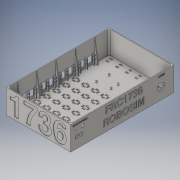
# Autodesk Inventor part: main_enclosure
Saved by Autodesk Inventor 2016 (Build 200138000, 138)
## iProperties
Created: 2015-08-24
Part Number: main_enclosure
Material: Generic
Document SubType Name: Modeling
Designer: Chris Gerth
Density: 1 g/cm^3
Appearance: Default
Sheet Metal Rule: Default
Author: Chris Gerth
Autodesk Inventor part; units mm, degrees
(part 1 of 3)
ref_plane "YZ Plane" through (0, 0, 0) normal (1, 0, 0) x (0, 1, 0)
ref_plane "XZ Plane" through (0, 0, 0) normal (0, 1, 0) x (-1, 0, 0)
ref_plane "XY Plane" through (0, 0, 0) normal (0, 0, 1) x (1, 0, 0)
sketch "Sketch1" plane through (0, 0, 0) normal (0, 1, 0) x (-1, 0, 0)
  line L0 (127, 203.2) -> (-127, 203.2)
  line L1 (-127, 203.2) -> (-127, -203.2)
  line L2 (-127, -203.2) -> (127, -203.2)
  line L3 (127, -203.2) -> (127, 203.2)
  line L4 (117.475, 184.15) -> (112.7125, 184.15)
  line L5 (112.7125, 184.15) -> (112.7125, 174.625)
  line L6 (112.7125, 174.625) -> (117.475, 174.625)
  line L7 (117.475, 174.625) -> (117.475, 184.15)
  line L8 (109.5375, 174.625) -> (100.0125, 174.625)
  line L9 (100.0125, 174.625) -> (100.0125, 169.8625)
  line L10 (100.0125, 169.8625) -> (109.5375, 169.8625)
  line L11 (109.5375, 169.8625) -> (109.5375, 174.625)
  line L12 (96.8375, 174.625) -> (92.0652, 174.625)
  line L13 (92.0652, 174.625) -> (92.0652, 184.2167)
  line L14 (92.0652, 184.2167) -> (96.8375, 184.2167)
  line L15 (96.8375, 184.2167) -> (96.8375, 174.625)
  line L16 (109.5375, 184.15) -> (100.0125, 184.15)
  line L17 (100.0125, 184.15) -> (100.0125, 188.9125)
  line L18 (100.0125, 188.9125) -> (109.5375, 188.9125)
  line L19 (109.5375, 188.9125) -> (109.5375, 184.15)
  line L20 (112.7125, 146.05) -> (112.7125, 136.525)
  line L21 (117.475, 146.05) -> (112.7125, 146.05)
  line L22 (112.7125, 136.525) -> (117.475, 136.525)
  line L23 (117.475, 136.525) -> (117.475, 146.05)
  line L24 (109.5375, 131.7625) -> (109.5375, 136.525)
  line L25 (109.5375, 150.8125) -> (109.5375, 146.05)
  line L26 (100.0125, 136.525) -> (100.0125, 131.7625)
  line L27 (100.0125, 131.7625) -> (109.5375, 131.7625)
  line L28 (100.0125, 146.05) -> (100.0125, 150.8125)
  line L29 (100.0125, 150.8125) -> (109.5375, 150.8125)
  line L30 (109.5375, 136.525) -> (100.0125, 136.525)
  line L31 (109.5375, 146.05) -> (100.0125, 146.05)
  line L32 (96.8375, 146.1167) -> (96.8375, 136.525)
  line L33 (96.8375, 136.525) -> (92.0652, 136.525)
  line L34 (92.0652, 136.525) -> (92.0652, 146.1167)
  line L35 (92.0652, 146.1167) -> (96.8375, 146.1167)
  line L36 (112.7125, 107.95) -> (112.7125, 98.425)
  line L37 (117.475, 107.95) -> (112.7125, 107.95)
  line L38 (112.7125, 98.425) -> (117.475, 98.425)
  line L39 (117.475, 98.425) -> (117.475, 107.95)
  line L40 (109.5375, 93.6625) -> (109.5375, 98.425)
  line L41 (109.5375, 112.7125) -> (109.5375, 107.95)
  line L42 (100.0125, 98.425) -> (100.0125, 93.6625)
  line L43 (100.0125, 93.6625) -> (109.5375, 93.6625)
  line L44 (100.0125, 107.95) -> (100.0125, 112.7125)
  line L45 (100.0125, 112.7125) -> (109.5375, 112.7125)
  line L46 (109.5375, 98.425) -> (100.0125, 98.425)
  line L47 (109.5375, 107.95) -> (100.0125, 107.95)
  line L48 (96.8375, 108.0167) -> (96.8375, 98.425)
  line L49 (96.8375, 98.425) -> (92.0652, 98.425)
  line L50 (92.0652, 98.425) -> (92.0652, 108.0167)
  line L51 (92.0652, 108.0167) -> (96.8375, 108.0167)
  line L52 (112.7125, 69.85) -> (112.7125, 60.325)
  line L53 (117.475, 69.85) -> (112.7125, 69.85)
  line L54 (112.7125, 60.325) -> (117.475, 60.325)
  line L55 (117.475, 60.325) -> (117.475, 69.85)
  line L56 (109.5375, 55.5625) -> (109.5375, 60.325)
  line L57 (109.5375, 74.6125) -> (109.5375, 69.85)
  line L58 (100.0125, 60.325) -> (100.0125, 55.5625)
  line L59 (100.0125, 55.5625) -> (109.5375, 55.5625)
  line L60 (100.0125, 69.85) -> (100.0125, 74.6125)
  line L61 (100.0125, 74.6125) -> (109.5375, 74.6125)
  line L62 (109.5375, 60.325) -> (100.0125, 60.325)
  line L63 (109.5375, 69.85) -> (100.0125, 69.85)
  line L64 (96.8375, 69.9167) -> (96.8375, 60.325)
  line L65 (96.8375, 60.325) -> (92.0652, 60.325)
  line L66 (92.0652, 60.325) -> (92.0652, 69.9167)
  line L67 (92.0652, 69.9167) -> (96.8375, 69.9167)
  line L68 (112.7125, 31.75) -> (112.7125, 22.225)
  line L69 (117.475, 31.75) -> (112.7125, 31.75)
  line L70 (112.7125, 22.225) -> (117.475, 22.225)
  line L71 (117.475, 22.225) -> (117.475, 31.75)
  line L72 (109.5375, 17.4625) -> (109.5375, 22.225)
  line L73 (109.5375, 36.5125) -> (109.5375, 31.75)
  line L74 (100.0125, 22.225) -> (100.0125, 17.4625)
  line L75 (100.0125, 17.4625) -> (109.5375, 17.4625)
  line L76 (100.0125, 31.75) -> (100.0125, 36.5125)
  line L77 (100.0125, 36.5125) -> (109.5375, 36.5125)
  line L78 (109.5375, 22.225) -> (100.0125, 22.225)
  line L79 (109.5375, 31.75) -> (100.0125, 31.75)
  line L80 (96.8375, 31.8167) -> (96.8375, 22.225)
  line L81 (96.8375, 22.225) -> (92.0652, 22.225)
  line L82 (92.0652, 22.225) -> (92.0652, 31.8167)
  line L83 (92.0652, 31.8167) -> (96.8375, 31.8167)
  line L84 (112.7125, -6.35) -> (112.7125, -15.875)
  line L85 (117.475, -6.35) -> (112.7125, -6.35)
  line L86 (112.7125, -15.875) -> (117.475, -15.875)
  line L87 (117.475, -15.875) -> (117.475, -6.35)
  line L88 (109.5375, -20.6375) -> (109.5375, -15.875)
  line L89 (109.5375, -1.5875) -> (109.5375, -6.35)
  line L90 (100.0125, -15.875) -> (100.0125, -20.6375)
  line L91 (100.0125, -20.6375) -> (109.5375, -20.6375)
  line L92 (100.0125, -6.35) -> (100.0125, -1.5875)
  line L93 (100.0125, -1.5875) -> (109.5375, -1.5875)
  line L94 (109.5375, -15.875) -> (100.0125, -15.875)
  line L95 (109.5375, -6.35) -> (100.0125, -6.35)
  line L96 (96.8375, -6.2833) -> (96.8375, -15.875)
  line L97 (96.8375, -15.875) -> (92.0652, -15.875)
  line L98 (92.0652, -15.875) -> (92.0652, -6.2833)
  line L99 (92.0652, -6.2833) -> (96.8375, -6.2833)
  line L100 (112.7125, -44.45) -> (112.7125, -53.975)
  line L101 (117.475, -44.45) -> (112.7125, -44.45)
  line L102 (112.7125, -53.975) -> (117.475, -53.975)
  line L103 (117.475, -53.975) -> (117.475, -44.45)
  line L104 (109.5375, -58.7375) -> (109.5375, -53.975)
  line L105 (109.5375, -39.6875) -> (109.5375, -44.45)
  line L106 (100.0125, -53.975) -> (100.0125, -58.7375)
  line L107 (100.0125, -58.7375) -> (109.5375, -58.7375)
  line L108 (100.0125, -44.45) -> (100.0125, -39.6875)
  line L109 (100.0125, -39.6875) -> (109.5375, -39.6875)
  line L110 (109.5375, -53.975) -> (100.0125, -53.975)
  line L111 (109.5375, -44.45) -> (100.0125, -44.45)
  line L112 (96.8375, -44.3833) -> (96.8375, -53.975)
  line L113 (96.8375, -53.975) -> (92.0652, -53.975)
  line L114 (92.0652, -53.975) -> (92.0652, -44.3833)
  line L115 (92.0652, -44.3833) -> (96.8375, -44.3833)
  line L116 (74.6125, 184.15) -> (74.6125, 174.625)
  line L117 (79.375, 184.15) -> (74.6125, 184.15)
  line L118 (74.6125, 174.625) -> (79.375, 174.625)
  line L119 (79.375, 174.625) -> (79.375, 184.15)
  line L120 (71.4375, 169.8625) -> (71.4375, 174.625)
  line L121 (71.4375, 188.9125) -> (71.4375, 184.15)
  line L122 (61.9125, 174.625) -> (61.9125, 169.8625)
  line L123 (61.9125, 169.8625) -> (71.4375, 169.8625)
  line L124 (61.9125, 184.15) -> (61.9125, 188.9125)
  line L125 (61.9125, 188.9125) -> (71.4375, 188.9125)
  line L126 (71.4375, 174.625) -> (61.9125, 174.625)
  line L127 (71.4375, 184.15) -> (61.9125, 184.15)
  line L128 (58.7375, 184.2167) -> (58.7375, 174.625)
  line L129 (58.7375, 174.625) -> (53.9652, 174.625)
  line L130 (53.9652, 174.625) -> (53.9652, 184.2167)
  line L131 (53.9652, 184.2167) -> (58.7375, 184.2167)
  line L132 (74.6125, 146.05) -> (74.6125, 136.525)
  line L133 (79.375, 146.05) -> (74.6125, 146.05)
  line L134 (74.6125, 136.525) -> (79.375, 136.525)
  line L135 (79.375, 136.525) -> (79.375, 146.05)
  line L136 (71.4375, 131.7625) -> (71.4375, 136.525)
  line L137 (71.4375, 150.8125) -> (71.4375, 146.05)
  line L138 (61.9125, 136.525) -> (61.9125, 131.7625)
  line L139 (61.9125, 131.7625) -> (71.4375, 131.7625)
  line L140 (61.9125, 146.05) -> (61.9125, 150.8125)
  line L141 (61.9125, 150.8125) -> (71.4375, 150.8125)
  line L142 (71.4375, 136.525) -> (61.9125, 136.525)
  line L143 (71.4375, 146.05) -> (61.9125, 146.05)
  line L144 (58.7375, 146.1167) -> (58.7375, 136.525)
  line L145 (58.7375, 136.525) -> (53.9652, 136.525)
  line L146 (53.9652, 136.525) -> (53.9652, 146.1167)
  line L147 (53.9652, 146.1167) -> (58.7375, 146.1167)
  line L148 (74.6125, 107.95) -> (74.6125, 98.425)
  line L149 (79.375, 107.95) -> (74.6125, 107.95)
  line L150 (74.6125, 98.425) -> (79.375, 98.425)
  line L151 (79.375, 98.425) -> (79.375, 107.95)
  line L152 (71.4375, 93.6625) -> (71.4375, 98.425)
  line L153 (71.4375, 112.7125) -> (71.4375, 107.95)
  line L154 (61.9125, 98.425) -> (61.9125, 93.6625)
  line L155 (61.9125, 93.6625) -> (71.4375, 93.6625)
  line L156 (61.9125, 107.95) -> (61.9125, 112.7125)
  line L157 (61.9125, 112.7125) -> (71.4375, 112.7125)
  line L158 (71.4375, 98.425) -> (61.9125, 98.425)
  line L159 (71.4375, 107.95) -> (61.9125, 107.95)
  line L160 (58.7375, 108.0167) -> (58.7375, 98.425)
  line L161 (58.7375, 98.425) -> (53.9652, 98.425)
  line L162 (53.9652, 98.425) -> (53.9652, 108.0167)
  line L163 (53.9652, 108.0167) -> (58.7375, 108.0167)
  line L164 (74.6125, 69.85) -> (74.6125, 60.325)
  line L165 (79.375, 69.85) -> (74.6125, 69.85)
  line L166 (74.6125, 60.325) -> (79.375, 60.325)
  line L167 (79.375, 60.325) -> (79.375, 69.85)
  line L168 (71.4375, 55.5625) -> (71.4375, 60.325)
  line L169 (71.4375, 74.6125) -> (71.4375, 69.85)
  line L170 (61.9125, 60.325) -> (61.9125, 55.5625)
  line L171 (61.9125, 55.5625) -> (71.4375, 55.5625)
  line L172 (61.9125, 69.85) -> (61.9125, 74.6125)
  line L173 (61.9125, 74.6125) -> (71.4375, 74.6125)
  line L174 (71.4375, 60.325) -> (61.9125, 60.325)
  line L175 (71.4375, 69.85) -> (61.9125, 69.85)
  line L176 (58.7375, 69.9167) -> (58.7375, 60.325)
  line L177 (58.7375, 60.325) -> (53.9652, 60.325)
  line L178 (53.9652, 60.325) -> (53.9652, 69.9167)
  line L179 (53.9652, 69.9167) -> (58.7375, 69.9167)
  line L180 (74.6125, 31.75) -> (74.6125, 22.225)
  line L181 (79.375, 31.75) -> (74.6125, 31.75)
  line L182 (74.6125, 22.225) -> (79.375, 22.225)
  line L183 (79.375, 22.225) -> (79.375, 31.75)
  line L184 (71.4375, 17.4625) -> (71.4375, 22.225)
  line L185 (71.4375, 36.5125) -> (71.4375, 31.75)
  line L186 (61.9125, 22.225) -> (61.9125, 17.4625)
  line L187 (61.9125, 17.4625) -> (71.4375, 17.4625)
  line L188 (61.9125, 31.75) -> (61.9125, 36.5125)
  line L189 (61.9125, 36.5125) -> (71.4375, 36.5125)
  line L190 (71.4375, 22.225) -> (61.9125, 22.225)
  line L191 (71.4375, 31.75) -> (61.9125, 31.75)
  line L192 (58.7375, 31.8167) -> (58.7375, 22.225)
  line L193 (58.7375, 22.225) -> (53.9652, 22.225)
  line L194 (53.9652, 22.225) -> (53.9652, 31.8167)
  line L195 (53.9652, 31.8167) -> (58.7375, 31.8167)
  line L196 (74.6125, -6.35) -> (74.6125, -15.875)
  line L197 (79.375, -6.35) -> (74.6125, -6.35)
  line L198 (74.6125, -15.875) -> (79.375, -15.875)
  line L199 (79.375, -15.875) -> (79.375, -6.35)
  line L200 (71.4375, -20.6375) -> (71.4375, -15.875)
  line L201 (71.4375, -1.5875) -> (71.4375, -6.35)
  line L202 (61.9125, -15.875) -> (61.9125, -20.6375)
  line L203 (61.9125, -20.6375) -> (71.4375, -20.6375)
  line L204 (61.9125, -6.35) -> (61.9125, -1.5875)
  line L205 (61.9125, -1.5875) -> (71.4375, -1.5875)
  line L206 (71.4375, -15.875) -> (61.9125, -15.875)
  line L207 (71.4375, -6.35) -> (61.9125, -6.35)
  line L208 (58.7375, -6.2833) -> (58.7375, -15.875)
  line L209 (58.7375, -15.875) -> (53.9652, -15.875)
  line L210 (53.9652, -15.875) -> (53.9652, -6.2833)
  line L211 (53.9652, -6.2833) -> (58.7375, -6.2833)
  line L212 (74.6125, -44.45) -> (74.6125, -53.975)
  line L213 (79.375, -44.45) -> (74.6125, -44.45)
  line L214 (74.6125, -53.975) -> (79.375, -53.975)
  line L215 (79.375, -53.975) -> (79.375, -44.45)
  line L216 (71.4375, -58.7375) -> (71.4375, -53.975)
  line L217 (71.4375, -39.6875) -> (71.4375, -44.45)
  line L218 (61.9125, -53.975) -> (61.9125, -58.7375)
  line L219 (61.9125, -58.7375) -> (71.4375, -58.7375)
  line L220 (61.9125, -44.45) -> (61.9125, -39.6875)
  line L221 (61.9125, -39.6875) -> (71.4375, -39.6875)
  line L222 (71.4375, -53.975) -> (61.9125, -53.975)
  line L223 (71.4375, -44.45) -> (61.9125, -44.45)
  line L224 (58.7375, -44.3833) -> (58.7375, -53.975)
  line L225 (58.7375, -53.975) -> (53.9652, -53.975)
  line L226 (53.9652, -53.975) -> (53.9652, -44.3833)
  line L227 (53.9652, -44.3833) -> (58.7375, -44.3833)
  line L228 (36.5125, 184.15) -> (36.5125, 174.625)
  line L229 (41.275, 184.15) -> (36.5125, 184.15)
  line L230 (36.5125, 174.625) -> (41.275, 174.625)
  line L231 (41.275, 174.625) -> (41.275, 184.15)
  line L232 (33.3375, 169.8625) -> (33.3375, 174.625)
  line L233 (33.3375, 188.9125) -> (33.3375, 184.15)
  line L234 (23.8125, 174.625) -> (23.8125, 169.8625)
  line L235 (23.8125, 169.8625) -> (33.3375, 169.8625)
  line L236 (23.8125, 184.15) -> (23.8125, 188.9125)
  line L237 (23.8125, 188.9125) -> (33.3375, 188.9125)
  line L238 (33.3375, 174.625) -> (23.8125, 174.625)
  line L239 (33.3375, 184.15) -> (23.8125, 184.15)
  line L240 (20.6375, 184.2167) -> (20.6375, 174.625)
  line L241 (20.6375, 174.625) -> (15.8652, 174.625)
  line L242 (15.8652, 174.625) -> (15.8652, 184.2167)
  line L243 (15.8652, 184.2167) -> (20.6375, 184.2167)
  line L244 (36.5125, 146.05) -> (36.5125, 136.525)
  line L245 (41.275, 146.05) -> (36.5125, 146.05)
  line L246 (36.5125, 136.525) -> (41.275, 136.525)
  line L247 (41.275, 136.525) -> (41.275, 146.05)
  line L248 (33.3375, 131.7625) -> (33.3375, 136.525)
  line L249 (33.3375, 150.8125) -> (33.3375, 146.05)
  line L250 (23.8125, 136.525) -> (23.8125, 131.7625)
  line L251 (23.8125, 131.7625) -> (33.3375, 131.7625)
  line L252 (23.8125, 146.05) -> (23.8125, 150.8125)
  line L253 (23.8125, 150.8125) -> (33.3375, 150.8125)
  line L254 (33.3375, 136.525) -> (23.8125, 136.525)
  line L255 (33.3375, 146.05) -> (23.8125, 146.05)
  line L256 (20.6375, 146.1167) -> (20.6375, 136.525)
  line L257 (20.6375, 136.525) -> (15.8652, 136.525)
  line L258 (15.8652, 136.525) -> (15.8652, 146.1167)
  line L259 (15.8652, 146.1167) -> (20.6375, 146.1167)
  line L260 (36.5125, 107.95) -> (36.5125, 98.425)
  line L261 (41.275, 107.95) -> (36.5125, 107.95)
  line L262 (36.5125, 98.425) -> (41.275, 98.425)
  line L263 (41.275, 98.425) -> (41.275, 107.95)
  line L264 (33.3375, 93.6625) -> (33.3375, 98.425)
  line L265 (33.3375, 112.7125) -> (33.3375, 107.95)
  line L266 (23.8125, 98.425) -> (23.8125, 93.6625)
  line L267 (23.8125, 93.6625) -> (33.3375, 93.6625)
  line L268 (23.8125, 107.95) -> (23.8125, 112.7125)
  line L269 (23.8125, 112.7125) -> (33.3375, 112.7125)
  line L270 (33.3375, 98.425) -> (23.8125, 98.425)
  line L271 (33.3375, 107.95) -> (23.8125, 107.95)
  line L272 (20.6375, 108.0167) -> (20.6375, 98.425)
  line L273 (20.6375, 98.425) -> (15.8652, 98.425)
  line L274 (15.8652, 98.425) -> (15.8652, 108.0167)
  line L275 (15.8652, 108.0167) -> (20.6375, 108.0167)
  line L276 (36.5125, 69.85) -> (36.5125, 60.325)
  line L277 (41.275, 69.85) -> (36.5125, 69.85)
  line L278 (36.5125, 60.325) -> (41.275, 60.325)
  line L279 (41.275, 60.325) -> (41.275, 69.85)
  line L280 (33.3375, 55.5625) -> (33.3375, 60.325)
  line L281 (33.3375, 74.6125) -> (33.3375, 69.85)
  line L282 (23.8125, 60.325) -> (23.8125, 55.5625)
  line L283 (23.8125, 55.5625) -> (33.3375, 55.5625)
  line L284 (23.8125, 69.85) -> (23.8125, 74.6125)
  line L285 (23.8125, 74.6125) -> (33.3375, 74.6125)
  line L286 (33.3375, 60.325) -> (23.8125, 60.325)
  line L287 (33.3375, 69.85) -> (23.8125, 69.85)
  line L288 (20.6375, 69.9167) -> (20.6375, 60.325)
  line L289 (20.6375, 60.325) -> (15.8652, 60.325)
  line L290 (15.8652, 60.325) -> (15.8652, 69.9167)
  line L291 (15.8652, 69.9167) -> (20.6375, 69.9167)
  line L292 (36.5125, 31.75) -> (36.5125, 22.225)
  line L293 (41.275, 31.75) -> (36.5125, 31.75)
  line L294 (36.5125, 22.225) -> (41.275, 22.225)
  line L295 (41.275, 22.225) -> (41.275, 31.75)
  line L296 (33.3375, 17.4625) -> (33.3375, 22.225)
  line L297 (33.3375, 36.5125) -> (33.3375, 31.75)
  line L298 (23.8125, 22.225) -> (23.8125, 17.4625)
  line L299 (23.8125, 17.4625) -> (33.3375, 17.4625)
  line L300 (23.8125, 31.75) -> (23.8125, 36.5125)
  line L301 (23.8125, 36.5125) -> (33.3375, 36.5125)
  line L302 (33.3375, 22.225) -> (23.8125, 22.225)
  line L303 (33.3375, 31.75) -> (23.8125, 31.75)
  line L304 (20.6375, 31.8167) -> (20.6375, 22.225)
  line L305 (20.6375, 22.225) -> (15.8652, 22.225)
  line L306 (15.8652, 22.225) -> (15.8652, 31.8167)
  line L307 (15.8652, 31.8167) -> (20.6375, 31.8167)
  line L308 (36.5125, -6.35) -> (36.5125, -15.875)
  line L309 (41.275, -6.35) -> (36.5125, -6.35)
  line L310 (36.5125, -15.875) -> (41.275, -15.875)
  line L311 (41.275, -15.875) -> (41.275, -6.35)
  line L312 (33.3375, -20.6375) -> (33.3375, -15.875)
  line L313 (33.3375, -1.5875) -> (33.3375, -6.35)
  line L314 (23.8125, -15.875) -> (23.8125, -20.6375)
  line L315 (23.8125, -20.6375) -> (33.3375, -20.6375)
  line L316 (23.8125, -6.35) -> (23.8125, -1.5875)
  line L317 (23.8125, -1.5875) -> (33.3375, -1.5875)
  line L318 (33.3375, -15.875) -> (23.8125, -15.875)
  line L319 (33.3375, -6.35) -> (23.8125, -6.35)
  line L320 (20.6375, -6.2833) -> (20.6375, -15.875)
  line L321 (20.6375, -15.875) -> (15.8652, -15.875)
  line L322 (15.8652, -15.875) -> (15.8652, -6.2833)
  line L323 (15.8652, -6.2833) -> (20.6375, -6.2833)
  line L324 (36.5125, -44.45) -> (36.5125, -53.975)
  line L325 (41.275, -44.45) -> (36.5125, -44.45)
  line L326 (36.5125, -53.975) -> (41.275, -53.975)
  line L327 (41.275, -53.975) -> (41.275, -44.45)
  line L328 (33.3375, -58.7375) -> (33.3375, -53.975)
  line L329 (33.3375, -39.6875) -> (33.3375, -44.45)
  line L330 (23.8125, -53.975) -> (23.8125, -58.7375)
  line L331 (23.8125, -58.7375) -> (33.3375, -58.7375)
  line L332 (23.8125, -44.45) -> (23.8125, -39.6875)
  line L333 (23.8125, -39.6875) -> (33.3375, -39.6875)
  line L334 (33.3375, -53.975) -> (23.8125, -53.975)
  line L335 (33.3375, -44.45) -> (23.8125, -44.45)
  line L336 (20.6375, -44.3833) -> (20.6375, -53.975)
  line L337 (20.6375, -53.975) -> (15.8652, -53.975)
  line L338 (15.8652, -53.975) -> (15.8652, -44.3833)
  line L339 (15.8652, -44.3833) -> (20.6375, -44.3833)
  line L340 (-1.5875, 184.15) -> (-1.5875, 174.625)
  line L341 (3.175, 184.15) -> (-1.5875, 184.15)
  line L342 (-1.5875, 174.625) -> (3.175, 174.625)
  line L343 (3.175, 174.625) -> (3.175, 184.15)
  line L344 (-4.7625, 169.8625) -> (-4.7625, 174.625)
  line L345 (-4.7625, 188.9125) -> (-4.7625, 184.15)
  line L346 (-14.2875, 174.625) -> (-14.2875, 169.8625)
  line L347 (-14.2875, 169.8625) -> (-4.7625, 169.8625)
  line L348 (-14.2875, 184.15) -> (-14.2875, 188.9125)
  line L349 (-14.2875, 188.9125) -> (-4.7625, 188.9125)
  line L350 (-4.7625, 174.625) -> (-14.2875, 174.625)
  line L351 (-4.7625, 184.15) -> (-14.2875, 184.15)
  line L352 (-17.4625, 184.2167) -> (-17.4625, 174.625)
  line L353 (-17.4625, 174.625) -> (-22.2348, 174.625)
  line L354 (-22.2348, 174.625) -> (-22.2348, 184.2167)
  line L355 (-22.2348, 184.2167) -> (-17.4625, 184.2167)
  line L356 (-1.5875, 146.05) -> (-1.5875, 136.525)
  line L357 (3.175, 146.05) -> (-1.5875, 146.05)
  line L358 (-1.5875, 136.525) -> (3.175, 136.525)
  line L359 (3.175, 136.525) -> (3.175, 146.05)
  line L360 (-4.7625, 131.7625) -> (-4.7625, 136.525)
  line L361 (-4.7625, 150.8125) -> (-4.7625, 146.05)
  line L362 (-14.2875, 136.525) -> (-14.2875, 131.7625)
  line L363 (-14.2875, 131.7625) -> (-4.7625, 131.7625)
  line L364 (-14.2875, 146.05) -> (-14.2875, 150.8125)
  line L365 (-14.2875, 150.8125) -> (-4.7625, 150.8125)
  line L366 (-4.7625, 136.525) -> (-14.2875, 136.525)
  line L367 (-4.7625, 146.05) -> (-14.2875, 146.05)
  line L368 (-17.4625, 146.1167) -> (-17.4625, 136.525)
  line L369 (-17.4625, 136.525) -> (-22.2348, 136.525)
  line L370 (-22.2348, 136.525) -> (-22.2348, 146.1167)
  line L371 (-22.2348, 146.1167) -> (-17.4625, 146.1167)
  line L372 (-1.5875, 107.95) -> (-1.5875, 98.425)
  line L373 (3.175, 107.95) -> (-1.5875, 107.95)
  line L374 (-1.5875, 98.425) -> (3.175, 98.425)
  line L375 (3.175, 98.425) -> (3.175, 107.95)
  line L376 (-4.7625, 93.6625) -> (-4.7625, 98.425)
  line L377 (-4.7625, 112.7125) -> (-4.7625, 107.95)
  line L378 (-14.2875, 98.425) -> (-14.2875, 93.6625)
  line L379 (-14.2875, 93.6625) -> (-4.7625, 93.6625)
  line L380 (-14.2875, 107.95) -> (-14.2875, 112.7125)
  line L381 (-14.2875, 112.7125) -> (-4.7625, 112.7125)
  line L382 (-4.7625, 98.425) -> (-14.2875, 98.425)
  line L383 (-4.7625, 107.95) -> (-14.2875, 107.95)
  line L384 (-17.4625, 108.0167) -> (-17.4625, 98.425)
  line L385 (-17.4625, 98.425) -> (-22.2348, 98.425)
  line L386 (-22.2348, 98.425) -> (-22.2348, 108.0167)
  line L387 (-22.2348, 108.0167) -> (-17.4625, 108.0167)
  line L388 (-1.5875, 69.85) -> (-1.5875, 60.325)
  line L389 (3.175, 69.85) -> (-1.5875, 69.85)
  line L390 (-1.5875, 60.325) -> (3.175, 60.325)
  line L391 (3.175, 60.325) -> (3.175, 69.85)
  line L392 (-4.7625, 55.5625) -> (-4.7625, 60.325)
  line L393 (-4.7625, 74.6125) -> (-4.7625, 69.85)
  line L394 (-14.2875, 60.325) -> (-14.2875, 55.5625)
  line L395 (-14.2875, 55.5625) -> (-4.7625, 55.5625)
  line L396 (-14.2875, 69.85) -> (-14.2875, 74.6125)
  line L397 (-14.2875, 74.6125) -> (-4.7625, 74.6125)
  line L398 (-4.7625, 60.325) -> (-14.2875, 60.325)
  line L399 (-4.7625, 69.85) -> (-14.2875, 69.85)
  line L400 (-17.4625, 69.9167) -> (-17.4625, 60.325)
  line L401 (-17.4625, 60.325) -> (-22.2348, 60.325)
  line L402 (-22.2348, 60.325) -> (-22.2348, 69.9167)
  line L403 (-22.2348, 69.9167) -> (-17.4625, 69.9167)
  line L404 (-1.5875, 31.75) -> (-1.5875, 22.225)
  line L405 (3.175, 31.75) -> (-1.5875, 31.75)
  line L406 (-1.5875, 22.225) -> (3.175, 22.225)
  line L407 (3.175, 22.225) -> (3.175, 31.75)
  line L408 (-4.7625, 17.4625) -> (-4.7625, 22.225)
  line L409 (-4.7625, 36.5125) -> (-4.7625, 31.75)
  line L410 (-14.2875, 22.225) -> (-14.2875, 17.4625)
  line L411 (-14.2875, 17.4625) -> (-4.7625, 17.4625)
  line L412 (-14.2875, 31.75) -> (-14.2875, 36.5125)
  line L413 (-14.2875, 36.5125) -> (-4.7625, 36.5125)
  line L414 (-4.7625, 22.225) -> (-14.2875, 22.225)
  line L415 (-4.7625, 31.75) -> (-14.2875, 31.75)
  line L416 (-17.4625, 31.8167) -> (-17.4625, 22.225)
  line L417 (-17.4625, 22.225) -> (-22.2348, 22.225)
  line L418 (-22.2348, 22.225) -> (-22.2348, 31.8167)
  line L419 (-22.2348, 31.8167) -> (-17.4625, 31.8167)
  line L420 (-1.5875, -6.35) -> (-1.5875, -15.875)
  line L421 (3.175, -6.35) -> (-1.5875, -6.35)
  line L422 (-1.5875, -15.875) -> (3.175, -15.875)
  line L423 (3.175, -15.875) -> (3.175, -6.35)
  line L424 (-4.7625, -20.6375) -> (-4.7625, -15.875)
  line L425 (-4.7625, -1.5875) -> (-4.7625, -6.35)
  line L426 (-14.2875, -15.875) -> (-14.2875, -20.6375)
  line L427 (-14.2875, -20.6375) -> (-4.7625, -20.6375)
  line L428 (-14.2875, -6.35) -> (-14.2875, -1.5875)
  line L429 (-14.2875, -1.5875) -> (-4.7625, -1.5875)
  line L430 (-4.7625, -15.875) -> (-14.2875, -15.875)
  line L431 (-4.7625, -6.35) -> (-14.2875, -6.35)
  line L432 (-17.4625, -6.2833) -> (-17.4625, -15.875)
  line L433 (-17.4625, -15.875) -> (-22.2348, -15.875)
  line L434 (-22.2348, -15.875) -> (-22.2348, -6.2833)
  line L435 (-22.2348, -6.2833) -> (-17.4625, -6.2833)
  line L436 (-1.5875, -44.45) -> (-1.5875, -53.975)
  line L437 (3.175, -44.45) -> (-1.5875, -44.45)
  line L438 (-1.5875, -53.975) -> (3.175, -53.975)
  line L439 (3.175, -53.975) -> (3.175, -44.45)
  line L440 (-4.7625, -58.7375) -> (-4.7625, -53.975)
  line L441 (-4.7625, -39.6875) -> (-4.7625, -44.45)
  line L442 (-14.2875, -53.975) -> (-14.2875, -58.7375)
  line L443 (-14.2875, -58.7375) -> (-4.7625, -58.7375)
  line L444 (-14.2875, -44.45) -> (-14.2875, -39.6875)
  line L445 (-14.2875, -39.6875) -> (-4.7625, -39.6875)
  line L446 (-4.7625, -53.975) -> (-14.2875, -53.975)
  line L447 (-4.7625, -44.45) -> (-14.2875, -44.45)
  line L448 (-17.4625, -44.3833) -> (-17.4625, -53.975)
  line L449 (-17.4625, -53.975) -> (-22.2348, -53.975)
  line L450 (-22.2348, -53.975) -> (-22.2348, -44.3833)
  line L451 (-22.2348, -44.3833) -> (-17.4625, -44.3833)
  line L452 (-39.6875, 184.15) -> (-39.6875, 174.625)
  line L453 (-34.925, 184.15) -> (-39.6875, 184.15)
  line L454 (-39.6875, 174.625) -> (-34.925, 174.625)
  line L455 (-34.925, 174.625) -> (-34.925, 184.15)
  line L456 (-42.8625, 169.8625) -> (-42.8625, 174.625)
  line L457 (-42.8625, 188.9125) -> (-42.8625, 184.15)
  line L458 (-52.3875, 174.625) -> (-52.3875, 169.8625)
  line L459 (-52.3875, 169.8625) -> (-42.8625, 169.8625)
  line L460 (-52.3875, 184.15) -> (-52.3875, 188.9125)
  line L461 (-52.3875, 188.9125) -> (-42.8625, 188.9125)
  line L462 (-42.8625, 174.625) -> (-52.3875, 174.625)
  line L463 (-42.8625, 184.15) -> (-52.3875, 184.15)
  line L464 (-55.5625, 184.2167) -> (-55.5625, 174.625)
  line L465 (-55.5625, 174.625) -> (-60.3348, 174.625)
  line L466 (-60.3348, 174.625) -> (-60.3348, 184.2167)
  line L467 (-60.3348, 184.2167) -> (-55.5625, 184.2167)
  line L468 (-39.6875, 146.05) -> (-39.6875, 136.525)
  line L469 (-34.925, 146.05) -> (-39.6875, 146.05)
  line L470 (-39.6875, 136.525) -> (-34.925, 136.525)
  line L471 (-34.925, 136.525) -> (-34.925, 146.05)
  line L472 (-42.8625, 131.7625) -> (-42.8625, 136.525)
  line L473 (-42.8625, 150.8125) -> (-42.8625, 146.05)
  line L474 (-52.3875, 136.525) -> (-52.3875, 131.7625)
  line L475 (-52.3875, 131.7625) -> (-42.8625, 131.7625)
  line L476 (-52.3875, 146.05) -> (-52.3875, 150.8125)
  line L477 (-52.3875, 150.8125) -> (-42.8625, 150.8125)
  line L478 (-42.8625, 136.525) -> (-52.3875, 136.525)
  line L479 (-42.8625, 146.05) -> (-52.3875, 146.05)
  line L480 (-55.5625, 146.1167) -> (-55.5625, 136.525)
  line L481 (-55.5625, 136.525) -> (-60.3348, 136.525)
  line L482 (-60.3348, 136.525) -> (-60.3348, 146.1167)
  line L483 (-60.3348, 146.1167) -> (-55.5625, 146.1167)
  line L484 (-39.6875, 107.95) -> (-39.6875, 98.425)
  line L485 (-34.925, 107.95) -> (-39.6875, 107.95)
  line L486 (-39.6875, 98.425) -> (-34.925, 98.425)
  line L487 (-34.925, 98.425) -> (-34.925, 107.95)
  line L488 (-42.8625, 93.6625) -> (-42.8625, 98.425)
  line L489 (-42.8625, 112.7125) -> (-42.8625, 107.95)
  line L490 (-52.3875, 98.425) -> (-52.3875, 93.6625)
  line L491 (-52.3875, 93.6625) -> (-42.8625, 93.6625)
  line L492 (-52.3875, 107.95) -> (-52.3875, 112.7125)
  line L493 (-52.3875, 112.7125) -> (-42.8625, 112.7125)
  line L494 (-42.8625, 98.425) -> (-52.3875, 98.425)
  line L495 (-42.8625, 107.95) -> (-52.3875, 107.95)
  line L496 (-55.5625, 108.0167) -> (-55.5625, 98.425)
  line L497 (-55.5625, 98.425) -> (-60.3348, 98.425)
  line L498 (-60.3348, 98.425) -> (-60.3348, 108.0167)
  line L499 (-60.3348, 108.0167) -> (-55.5625, 108.0167)
  line L500 (-39.6875, 69.85) -> (-39.6875, 60.325)
  line L501 (-34.925, 69.85) -> (-39.6875, 69.85)
  line L502 (-39.6875, 60.325) -> (-34.925, 60.325)
  line L503 (-34.925, 60.325) -> (-34.925, 69.85)
  line L504 (-42.8625, 55.5625) -> (-42.8625, 60.325)
  line L505 (-42.8625, 74.6125) -> (-42.8625, 69.85)
  line L506 (-52.3875, 60.325) -> (-52.3875, 55.5625)
  line L507 (-52.3875, 55.5625) -> (-42.8625, 55.5625)
  line L508 (-52.3875, 69.85) -> (-52.3875, 74.6125)
  line L509 (-52.3875, 74.6125) -> (-42.8625, 74.6125)
  line L510 (-42.8625, 60.325) -> (-52.3875, 60.325)
  line L511 (-42.8625, 69.85) -> (-52.3875, 69.85)
  line L512 (-55.5625, 69.9167) -> (-55.5625, 60.325)
  line L513 (-55.5625, 60.325) -> (-60.3348, 60.325)
  line L514 (-60.3348, 60.325) -> (-60.3348, 69.9167)
  line L515 (-60.3348, 69.9167) -> (-55.5625, 69.9167)
  line L516 (-39.6875, 31.75) -> (-39.6875, 22.225)
  line L517 (-34.925, 31.75) -> (-39.6875, 31.75)
  line L518 (-39.6875, 22.225) -> (-34.925, 22.225)
  line L519 (-34.925, 22.225) -> (-34.925, 31.75)
  line L520 (-42.8625, 17.4625) -> (-42.8625, 22.225)
  line L521 (-42.8625, 36.5125) -> (-42.8625, 31.75)
  line L522 (-52.3875, 22.225) -> (-52.3875, 17.4625)
  line L523 (-52.3875, 17.4625) -> (-42.8625, 17.4625)
  line L524 (-52.3875, 31.75) -> (-52.3875, 36.5125)
  line L525 (-52.3875, 36.5125) -> (-42.8625, 36.5125)
  line L526 (-42.8625, 22.225) -> (-52.3875, 22.225)
  line L527 (-42.8625, 31.75) -> (-52.3875, 31.75)
  line L528 (-55.5625, 31.8167) -> (-55.5625, 22.225)
  line L529 (-55.5625, 22.225) -> (-60.3348, 22.225)
  line L530 (-60.3348, 22.225) -> (-60.3348, 31.8167)
  line L531 (-60.3348, 31.8167) -> (-55.5625, 31.8167)
  line L532 (-39.6875, -6.35) -> (-39.6875, -15.875)
  line L533 (-34.925, -6.35) -> (-39.6875, -6.35)
  line L534 (-39.6875, -15.875) -> (-34.925, -15.875)
  line L535 (-34.925, -15.875) -> (-34.925, -6.35)
  line L536 (-42.8625, -20.6375) -> (-42.8625, -15.875)
  line L537 (-42.8625, -1.5875) -> (-42.8625, -6.35)
  line L538 (-52.3875, -15.875) -> (-52.3875, -20.6375)
  line L539 (-52.3875, -20.6375) -> (-42.8625, -20.6375)
  line L540 (-52.3875, -6.35) -> (-52.3875, -1.5875)
  line L541 (-52.3875, -1.5875) -> (-42.8625, -1.5875)
  line L542 (-42.8625, -15.875) -> (-52.3875, -15.875)
  line L543 (-42.8625, -6.35) -> (-52.3875, -6.35)
  line L544 (-55.5625, -6.2833) -> (-55.5625, -15.875)
  line L545 (-55.5625, -15.875) -> (-60.3348, -15.875)
  line L546 (-60.3348, -15.875) -> (-60.3348, -6.2833)
  line L547 (-60.3348, -6.2833) -> (-55.5625, -6.2833)
  line L548 (-39.6875, -44.45) -> (-39.6875, -53.975)
  line L549 (-34.925, -44.45) -> (-39.6875, -44.45)
  line L550 (-39.6875, -53.975) -> (-34.925, -53.975)
  line L551 (-34.925, -53.975) -> (-34.925, -44.45)
  line L552 (-42.8625, -58.7375) -> (-42.8625, -53.975)
  line L553 (-42.8625, -39.6875) -> (-42.8625, -44.45)
  line L554 (-52.3875, -53.975) -> (-52.3875, -58.7375)
  line L555 (-52.3875, -58.7375) -> (-42.8625, -58.7375)
  line L556 (-52.3875, -44.45) -> (-52.3875, -39.6875)
  line L557 (-52.3875, -39.6875) -> (-42.8625, -39.6875)
  line L558 (-42.8625, -53.975) -> (-52.3875, -53.975)
  line L559 (-42.8625, -44.45) -> (-52.3875, -44.45)
  line L560 (-55.5625, -44.3833) -> (-55.5625, -53.975)
  line L561 (-55.5625, -53.975) -> (-60.3348, -53.975)
  line L562 (-60.3348, -53.975) -> (-60.3348, -44.3833)
  line L563 (-60.3348, -44.3833) -> (-55.5625, -44.3833)
  line L564 (-77.7875, 184.15) -> (-77.7875, 174.625)
  line L565 (-73.025, 184.15) -> (-77.7875, 184.15)
  line L566 (-77.7875, 174.625) -> (-73.025, 174.625)
  line L567 (-73.025, 174.625) -> (-73.025, 184.15)
  line L568 (-80.9625, 169.8625) -> (-80.9625, 174.625)
  line L569 (-80.9625, 188.9125) -> (-80.9625, 184.15)
  line L570 (-90.4875, 174.625) -> (-90.4875, 169.8625)
  line L571 (-90.4875, 169.8625) -> (-80.9625, 169.8625)
  line L572 (-90.4875, 184.15) -> (-90.4875, 188.9125)
  line L573 (-90.4875, 188.9125) -> (-80.9625, 188.9125)
  line L574 (-80.9625, 174.625) -> (-90.4875, 174.625)
  line L575 (-80.9625, 184.15) -> (-90.4875, 184.15)
  line L576 (-93.6625, 184.2167) -> (-93.6625, 174.625)
  line L577 (-93.6625, 174.625) -> (-98.4348, 174.625)
  line L578 (-98.4348, 174.625) -> (-98.4348, 184.2167)
  line L579 (-98.4348, 184.2167) -> (-93.6625, 184.2167)
  line L580 (-77.7875, 146.05) -> (-77.7875, 136.525)
  line L581 (-73.025, 146.05) -> (-77.7875, 146.05)
  line L582 (-77.7875, 136.525) -> (-73.025, 136.525)
  line L583 (-73.025, 136.525) -> (-73.025, 146.05)
  line L584 (-80.9625, 131.7625) -> (-80.9625, 136.525)
  line L585 (-80.9625, 150.8125) -> (-80.9625, 146.05)
  line L586 (-90.4875, 136.525) -> (-90.4875, 131.7625)
  line L587 (-90.4875, 131.7625) -> (-80.9625, 131.7625)
  line L588 (-90.4875, 146.05) -> (-90.4875, 150.8125)
  line L589 (-90.4875, 150.8125) -> (-80.9625, 150.8125)
  line L590 (-80.9625, 136.525) -> (-90.4875, 136.525)
  line L591 (-80.9625, 146.05) -> (-90.4875, 146.05)
  line L592 (-93.6625, 146.1167) -> (-93.6625, 136.525)
  line L593 (-93.6625, 136.525) -> (-98.4348, 136.525)
  line L594 (-98.4348, 136.525) -> (-98.4348, 146.1167)
  line L595 (-98.4348, 146.1167) -> (-93.6625, 146.1167)
  line L596 (-77.7875, 107.95) -> (-77.7875, 98.425)
  line L597 (-73.025, 107.95) -> (-77.7875, 107.95)
  line L598 (-77.7875, 98.425) -> (-73.025, 98.425)
  line L599 (-73.025, 98.425) -> (-73.025, 107.95)
  line L600 (-80.9625, 93.6625) -> (-80.9625, 98.425)
  line L601 (-80.9625, 112.7125) -> (-80.9625, 107.95)
  line L602 (-90.4875, 98.425) -> (-90.4875, 93.6625)
  line L603 (-90.4875, 93.6625) -> (-80.9625, 93.6625)
  line L604 (-90.4875, 107.95) -> (-90.4875, 112.7125)
  line L605 (-90.4875, 112.7125) -> (-80.9625, 112.7125)
  line L606 (-80.9625, 98.425) -> (-90.4875, 98.425)
  line L607 (-80.9625, 107.95) -> (-90.4875, 107.95)
  line L608 (-93.6625, 108.0167) -> (-93.6625, 98.425)
  line L609 (-93.6625, 98.425) -> (-98.4348, 98.425)
  line L610 (-98.4348, 98.425) -> (-98.4348, 108.0167)
  line L611 (-98.4348, 108.0167) -> (-93.6625, 108.0167)
  line L612 (-77.7875, 69.85) -> (-77.7875, 60.325)
  line L613 (-73.025, 69.85) -> (-77.7875, 69.85)
  line L614 (-77.7875, 60.325) -> (-73.025, 60.325)
  line L615 (-73.025, 60.325) -> (-73.025, 69.85)
  line L616 (-80.9625, 55.5625) -> (-80.9625, 60.325)
  line L617 (-80.9625, 74.6125) -> (-80.9625, 69.85)
  line L618 (-90.4875, 60.325) -> (-90.4875, 55.5625)
  line L619 (-90.4875, 55.5625) -> (-80.9625, 55.5625)
  line L620 (-90.4875, 69.85) -> (-90.4875, 74.6125)
  line L621 (-90.4875, 74.6125) -> (-80.9625, 74.6125)
  line L622 (-80.9625, 60.325) -> (-90.4875, 60.325)
  line L623 (-80.9625, 69.85) -> (-90.4875, 69.85)
  line L624 (-93.6625, 69.9167) -> (-93.6625, 60.325)
  line L625 (-93.6625, 60.325) -> (-98.4348, 60.325)
  line L626 (-98.4348, 60.325) -> (-98.4348, 69.9167)
  line L627 (-98.4348, 69.9167) -> (-93.6625, 69.9167)
  line L628 (-77.7875, 31.75) -> (-77.7875, 22.225)
  line L629 (-73.025, 31.75) -> (-77.7875, 31.75)
  line L630 (-77.7875, 22.225) -> (-73.025, 22.225)
  line L631 (-73.025, 22.225) -> (-73.025, 31.75)
  line L632 (-80.9625, 17.4625) -> (-80.9625, 22.225)
  line L633 (-80.9625, 36.5125) -> (-80.9625, 31.75)
  line L634 (-90.4875, 22.225) -> (-90.4875, 17.4625)
  line L635 (-90.4875, 17.4625) -> (-80.9625, 17.4625)
  line L636 (-90.4875, 31.75) -> (-90.4875, 36.5125)
  line L637 (-90.4875, 36.5125) -> (-80.9625, 36.5125)
  line L638 (-80.9625, 22.225) -> (-90.4875, 22.225)
  line L639 (-80.9625, 31.75) -> (-90.4875, 31.75)
  line L640 (-93.6625, 31.8167) -> (-93.6625, 22.225)
  line L641 (-93.6625, 22.225) -> (-98.4348, 22.225)
  line L642 (-98.4348, 22.225) -> (-98.4348, 31.8167)
  line L643 (-98.4348, 31.8167) -> (-93.6625, 31.8167)
  line L644 (-77.7875, -6.35) -> (-77.7875, -15.875)
  line L645 (-73.025, -6.35) -> (-77.7875, -6.35)
  line L646 (-77.7875, -15.875) -> (-73.025, -15.875)
  line L647 (-73.025, -15.875) -> (-73.025, -6.35)
  line L648 (-80.9625, -20.6375) -> (-80.9625, -15.875)
  line L649 (-80.9625, -1.5875) -> (-80.9625, -6.35)
  line L650 (-90.4875, -15.875) -> (-90.4875, -20.6375)
  line L651 (-90.4875, -20.6375) -> (-80.9625, -20.6375)
  line L652 (-90.4875, -6.35) -> (-90.4875, -1.5875)
  line L653 (-90.4875, -1.5875) -> (-80.9625, -1.5875)
  line L654 (-80.9625, -15.875) -> (-90.4875, -15.875)
  line L655 (-80.9625, -6.35) -> (-90.4875, -6.35)
  line L656 (-93.6625, -6.2833) -> (-93.6625, -15.875)
  line L657 (-93.6625, -15.875) -> (-98.4348, -15.875)
  line L658 (-98.4348, -15.875) -> (-98.4348, -6.2833)
  line L659 (-98.4348, -6.2833) -> (-93.6625, -6.2833)
  line L660 (-77.7875, -44.45) -> (-77.7875, -53.975)
  line L661 (-73.025, -44.45) -> (-77.7875, -44.45)
  line L662 (-77.7875, -53.975) -> (-73.025, -53.975)
  line L663 (-73.025, -53.975) -> (-73.025, -44.45)
  line L664 (-80.9625, -58.7375) -> (-80.9625, -53.975)
  line L665 (-80.9625, -39.6875) -> (-80.9625, -44.45)
  line L666 (-90.4875, -53.975) -> (-90.4875, -58.7375)
  line L667 (-90.4875, -58.7375) -> (-80.9625, -58.7375)
  line L668 (-90.4875, -44.45) -> (-90.4875, -39.6875)
  line L669 (-90.4875, -39.6875) -> (-80.9625, -39.6875)
  line L670 (-80.9625, -53.975) -> (-90.4875, -53.975)
  line L671 (-80.9625, -44.45) -> (-90.4875, -44.45)
  line L672 (-93.6625, -44.3833) -> (-93.6625, -53.975)
  line L673 (-93.6625, -53.975) -> (-98.4348, -53.975)
  line L674 (-98.4348, -53.975) -> (-98.4348, -44.3833)
  line L675 (-98.4348, -44.3833) -> (-93.6625, -44.3833)
  line L676 (109.5375, -190.5) -> (109.5375, -185.7375)
  line L677 (109.5375, -171.45) -> (109.5375, -176.2125)
  line L678 (100.0125, -185.7375) -> (100.0125, -190.5)
  line L679 (100.0125, -190.5) -> (109.5375, -190.5)
  line L680 (100.0125, -176.2125) -> (100.0125, -171.45)
  line L681 (100.0125, -171.45) -> (109.5375, -171.45)
  line L682 (109.5375, -185.7375) -> (100.0125, -185.7375)
  line L683 (109.5375, -176.2125) -> (100.0125, -176.2125)
  line L684 (71.4375, -185.7375) -> (61.9125, -185.7375)
  line L685 (61.9125, -185.7375) -> (61.9125, -190.5)
  line L686 (71.4375, -176.2125) -> (61.9125, -176.2125)
  line L687 (61.9125, -190.5) -> (71.4375, -190.5)
  line L688 (71.4375, -190.5) -> (71.4375, -185.7375)
  line L689 (61.9125, -171.45) -> (71.4375, -171.45)
  line L690 (61.9125, -176.2125) -> (61.9125, -171.45)
  line L691 (71.4375, -171.45) -> (71.4375, -176.2125)
  line L692 (33.3375, -185.7375) -> (23.8125, -185.7375)
  line L693 (23.8125, -185.7375) -> (23.8125, -190.5)
  line L694 (33.3375, -176.2125) -> (23.8125, -176.2125)
  line L695 (23.8125, -190.5) -> (33.3375, -190.5)
  line L696 (33.3375, -190.5) -> (33.3375, -185.7375)
  line L697 (23.8125, -171.45) -> (33.3375, -171.45)
  line L698 (23.8125, -176.2125) -> (23.8125, -171.45)
  line L699 (33.3375, -171.45) -> (33.3375, -176.2125)
  line L700 (-4.7625, -185.7375) -> (-14.2875, -185.7375)
  line L701 (-14.2875, -185.7375) -> (-14.2875, -190.5)
  line L702 (-4.7625, -176.2125) -> (-14.2875, -176.2125)
  line L703 (-14.2875, -190.5) -> (-4.7625, -190.5)
  line L704 (-4.7625, -190.5) -> (-4.7625, -185.7375)
  line L705 (-14.2875, -171.45) -> (-4.7625, -171.45)
  line L706 (-14.2875, -176.2125) -> (-14.2875, -171.45)
  line L707 (-4.7625, -171.45) -> (-4.7625, -176.2125)
  line L708 (-42.8625, -185.7375) -> (-52.3875, -185.7375)
  line L709 (-52.3875, -185.7375) -> (-52.3875, -190.5)
  line L710 (-42.8625, -176.2125) -> (-52.3875, -176.2125)
  line L711 (-52.3875, -190.5) -> (-42.8625, -190.5)
  line L712 (-42.8625, -190.5) -> (-42.8625, -185.7375)
  line L713 (-52.3875, -171.45) -> (-42.8625, -171.45)
  line L714 (-52.3875, -176.2125) -> (-52.3875, -171.45)
  line L715 (-42.8625, -171.45) -> (-42.8625, -176.2125)
  line L716 (-80.9625, -185.7375) -> (-90.4875, -185.7375)
  line L717 (-90.4875, -185.7375) -> (-90.4875, -190.5)
  line L718 (-80.9625, -176.2125) -> (-90.4875, -176.2125)
  line L719 (-90.4875, -190.5) -> (-80.9625, -190.5)
  line L720 (-80.9625, -190.5) -> (-80.9625, -185.7375)
  line L721 (-90.4875, -171.45) -> (-80.9625, -171.45)
  line L722 (-90.4875, -176.2125) -> (-90.4875, -171.45)
  line L723 (-80.9625, -171.45) -> (-80.9625, -176.2125)
  point P0 (0, 0)
  dimension "d0" = 254
  dimension "d1" = 406.4
  dimension "d4" = 38.1
  dimension "d7" = 38.1
  dimension "d16" = 38.1
  constraints: 1448 end point, 42 point on line, 10 parallel, 7 horizontal, 5 perpendicular, 3 collinear, 1 vertical, 1389 other
  measures "d0" distance of L2.end L1.end
  measures "d1" distance of L1.end L0.end
  measures "d4" distance of L5.end L20.end
  measures "d7" distance of L5.end L116.end
  measures "d16" distance of L678.end L685.end
extrude "Extrusion1" add sketch "Sketch1" along normal blind 5.08
sketch "Sketch2" plane through (0, 5.08, 0) normal (0, 1, 0) x (1, 0, 0)
  line L0 (-127, -203.2) -> (127, -203.2) projected
  line L1 (-127, -203.2) -> (127, -203.2)
  line L2 (127, -203.2) -> (127, 203.2)
  line L3 (127, 203.2) -> (-127, 203.2)
  line L4 (-127, 203.2) -> (-127, -203.2)
  line L5 (-123.825, -200.025) -> (123.825, -200.025)
  line L6 (123.825, -200.025) -> (123.825, 200.025)
  line L7 (123.825, 200.025) -> (-123.825, 200.025)
  line L8 (-123.825, 200.025) -> (-123.825, -200.025)
  point P0 (0, 0)
  constraints: 16 end point, 4 parallel, 2 horizontal, 2 perpendicular
extrude "Extrusion2" add sketch "Sketch2" along normal blind 88.9
sketch "Sketch3" plane through (0, 5.08, 0) normal (0, 1, 0) x (1, 0, 0)
  line L0 (-123.825, -163.5125) -> (-111.125, -163.5125)
  line L1 (-111.125, -163.5125) -> (-111.125, -160.3375)
  line L2 (-111.125, -160.3375) -> (-123.825, -160.3375)
  line L3 (-123.825, -160.3375) -> (-123.825, -163.5125)
  line L4 (111.1356, -130.1866) -> (123.8356, -130.1866)
  line L5 (123.8356, -130.1866) -> (123.8356, -127.0116)
  line L6 (123.8356, -127.0116) -> (111.1356, -127.0116)
  line L7 (111.1356, -127.0116) -> (111.1356, -130.1866)
  line L8 (-123.825, -87.3125) -> (-111.125, -87.3125)
  line L9 (-111.125, -87.3125) -> (-111.125, -84.1375)
  line L10 (-111.125, -84.1375) -> (-123.825, -84.1375)
  line L11 (-123.825, -84.1375) -> (-123.825, -87.3125)
  line L12 (111.125, -87.3125) -> (123.825, -87.3125)
  line L13 (123.825, -87.3125) -> (123.825, -84.1375)
  line L14 (123.825, -84.1375) -> (111.125, -84.1375)
  line L15 (111.125, -84.1375) -> (111.125, -87.3125)
  line L16 (-123.825, -11.1125) -> (-111.125, -11.1125)
  line L17 (-111.125, -11.1125) -> (-111.125, -7.9375)
  line L18 (-111.125, -7.9375) -> (-123.825, -7.9375)
  line L19 (-123.825, -7.9375) -> (-123.825, -11.1125)
  line L20 (111.125, -11.1125) -> (123.825, -11.1125)
  line L21 (123.825, -11.1125) -> (123.825, -7.9375)
  line L22 (123.825, -7.9375) -> (111.125, -7.9375)
  line L23 (111.125, -7.9375) -> (111.125, -11.1125)
  line L24 (-123.825, 65.0875) -> (-111.125, 65.0875)
  line L25 (-111.125, 65.0875) -> (-111.125, 68.2625)
  line L26 (-111.125, 68.2625) -> (-123.825, 68.2625)
  line L27 (-123.825, 68.2625) -> (-123.825, 65.0875)
  line L28 (111.125, 65.0875) -> (123.825, 65.0875)
  line L29 (123.825, 65.0875) -> (123.825, 68.2625)
  line L30 (123.825, 68.2625) -> (111.125, 68.2625)
  line L31 (111.125, 68.2625) -> (111.125, 65.0875)
  line L32 (-123.825, 141.2875) -> (-111.125, 141.2875)
  line L33 (-111.125, 141.2875) -> (-111.125, 144.4625)
  line L34 (-111.125, 144.4625) -> (-123.825, 144.4625)
  line L35 (-123.825, 144.4625) -> (-123.825, 141.2875)
  line L36 (111.125, 114.3339) -> (123.825, 114.3339)
  line L37 (123.825, 114.3339) -> (123.825, 117.5089)
  line L38 (123.825, 117.5089) -> (111.125, 117.5089)
  line L39 (111.125, 117.5089) -> (111.125, 114.3339)
  line L40 (-123.825, 200.025) -> (-123.825, -200.025) projected
  line L41 (-123.825, -200.025) -> (-117.475, -200.025)
  line L42 (-123.825, -200.025) -> (123.825, -200.025) projected
  line L43 (-123.825, -193.675) -> (-117.475, -200.025)
  line L44 (-123.825, -193.675) -> (-123.825, -200.025)
  line L45 (-123.825, -200.025) -> (-117.475, -200.025)
  line L46 (-123.825, 193.675) -> (-117.475, 200.025)
  line L47 (123.825, 200.025) -> (-123.825, 200.025) projected
  line L48 (-117.475, 200.025) -> (-123.825, 200.025)
  line L49 (-123.825, 200.025) -> (-123.825, 193.675)
  line L50 (123.825, 193.4089) -> (117.475, 200.025)
  line L51 (117.475, 200.025) -> (123.825, 200.025)
  line L52 (123.825, 200.025) -> (123.825, 193.4089)
  line L53 (117.475, -200.025) -> (123.825, -193.9304)
  line L54 (123.825, -200.025) -> (123.825, 200.025) projected
  line L55 (123.825, -193.9304) -> (123.825, -200.025)
  point P0 (0, 0)
  dimension "d27" = 237.3122
  dimension "d30" = 76.2
  constraints: 104 end point, 7 point on line, 5 collinear, 5 perpendicular, 2 horizontal, 2 parallel, 2 vertical, 47 other
  measures "d27" distance of L0.start L4.start
  measures "d30" distance of L0.start L8.start
extrude "Extrusion3" add sketch "Sketch3" along normal blind 88.9 contours L3 L2 L1 L0 | L43 L41 L40 | L11 L10 L9 L8 | L53 L54 L42 | L19 L18 L17 L16 | L54 L6 L5 L4 | L4 L7 L6 L54 | L27 L26 L25 L24 | L12 L15 L14 L13 | L35 L34 L33 L32 | L20 L23 L22 L21 | L40 L47 L46 | L28 L31 L30 L29 | L47 L52 L50 | L36 L39 L38 L37
chamfer "Chamfer1" distance 12.7 distance2 88.9 1 edges at (-111.125, 93.98, -142.875) measured on face at (-125.9417, 93.98, 53.4458)
chamfer "Chamfer2" distance 12.7 distance2 88.9 1 edges at (-111.125, 93.98, -66.675) measured on face at (-125.9417, 93.98, 53.4458)
chamfer "Chamfer3" distance 12.7 distance2 88.9 1 edges at (-111.125, 93.98, 9.525) measured on face at (-125.9417, 93.98, 53.4458)
chamfer "Chamfer4" distance 12.7 distance2 88.9 1 edges at (-111.125, 93.98, 85.725) measured on face at (-125.9417, 93.98, 53.4458)
chamfer "Chamfer5" distance 12.7 distance2 88.9 1 edges at (-111.125, 93.98, 161.925) measured on face at (-125.9417, 93.98, 53.4458)
chamfer "Chamfer6" distance 12.7 distance2 88.9 1 edges at (111.125, 93.98, -115.9214) measured on face at (-125.9417, 93.98, 53.4458)
chamfer "Chamfer7" distance 12.7 distance2 88.9 1 edges at (111.125, 93.98, -66.675) measured on face at (-125.9417, 93.98, 53.4458)
chamfer "Chamfer8" distance 12.7 distance2 88.9 1 edges at (111.125, 93.98, 9.525) measured on face at (-125.9417, 93.98, 53.4458)
chamfer "Chamfer9" distance 12.7 distance2 88.9 1 edges at (111.125, 93.98, 85.725) measured on face at (-125.9417, 93.98, 53.4458)
sketch "Sketch6" plane through (0, 5.08, 0) normal (0, 1, 0) x (1, 0, 0)
  circle A0 centre (-54.5952, 80.5731) radius 2.9957
  circle A1 centre (-53.4649, 128.8906) radius 2.9957
  circle A2 centre (-2.5479, 85.8287) radius 2.9957
  circle A3 centre (-2.5479, 113.8585) radius 2.9957
  point P0 (0, 0)
  constraints: 4 centre point
extrude "Extrusion4" add sketch "Sketch6" along normal blind 6.35